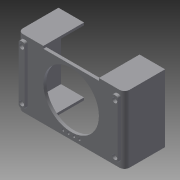
# Autodesk Inventor part: Enclosure01
Saved by Autodesk Inventor 2013 (Build 170138000, 138)
## iProperties
Created: 2014-04-13
Part Number: Enclosure01
Material: Generic
Document SubType Name: Modeling
Designer: spichelh
Density: 1 g/cm^3
Author: spichelh
Autodesk Inventor part; units mm, degrees
ref_plane "YZ Plane" through (0, 0, 0) normal (1, 0, 0) x (0, 1, 0)
ref_plane "XZ Plane" through (0, 0, 0) normal (0, 1, 0) x (-1, 0, 0)
ref_plane "XY Plane" through (0, 0, 0) normal (0, 0, 1) x (1, 0, 0)
sketch "Sketch1" plane through (0, 0, 0) normal (0, 0, 1) x (1, 0, 0)
  circle A0 centre (37.2069, 31.0185) radius 28
  line L0 (-13.5931, 3.1035) -> (88.0069, 3.1035) construction
  line L1 (14.2069, 60.2535) -> (-13.5931, 60.2535) construction
  line L2 (88.0069, 60.2535) -> (60.0869, 60.2535) construction
  line L3 (88.0069, 3.1035) -> (88.0069, 60.2535) construction
  line L4 (-13.5931, 60.2535) -> (-13.5931, 3.1035) construction
  line L5 (11.269, 60.2207) -> (67.149, 60.2207) construction
  line L6 (67.149, 60.2207) -> (67.149, 72.2207) construction
  line L7 (67.149, 72.2207) -> (11.269, 72.2207) construction
  line L8 (11.269, 72.2207) -> (11.269, 60.2207) construction
  circle A1 centre (61.389, 6.2635) radius 1.5 construction
  circle A2 centre (61.389, 55.7935) radius 1.5 construction
  circle A3 centre (5.509, 55.7935) radius 1.5 construction
  circle A4 centre (11.269, 6.9135) radius 1.5 construction
  arc A5 (11.269, 7.6907) -> (11.269, 1.6907) centre (11.269, 4.6907) ccw construction
  line L9 (11.269, 1.6907) -> (11.269, -3.7465) construction
  line L10 (11.269, -3.7465) -> (67.149, -3.7465) construction
  line L11 (67.149, -3.7465) -> (67.149, 1.6907) construction
  arc A6 (67.149, 1.6907) -> (67.149, 7.6907) centre (67.149, 4.6907) ccw construction
  line L12 (67.149, 7.6907) -> (67.149, 51.2207) construction
  arc A7 (67.149, 51.2207) -> (67.149, 57.2207) centre (67.149, 54.2207) ccw construction
  line L13 (67.149, 57.2207) -> (67.149, 60.2207) construction
  line L14 (67.149, 60.2207) -> (11.269, 60.2207) construction
  line L15 (11.269, 60.2207) -> (11.269, 57.2207) construction
  arc A8 (11.269, 57.2207) -> (11.269, 51.2207) centre (11.269, 54.2207) ccw construction
  line L16 (11.269, 51.2207) -> (11.269, 7.6907) construction
  line L17 (-16.5931, -3.7465) -> (91.0069, -3.7465)
  line L18 (91.0069, -3.7465) -> (91.0069, 64.2535)
  line L19 (91.0069, 64.2535) -> (-16.5931, 64.2535)
  line L20 (-16.5931, 64.2535) -> (-16.5931, -3.7465)
  line L21 (37.2069, -3.7465) -> (37.2069, 64.2535) construction
  circle A9 centre (37.2069, 31.0185) radius 23 projected
  point P0 (0, 0)
  dimension "d42" = 0
  dimension "d43" = 3
  dimension "d44" = 3
  dimension "d45" = 4
  dimension "d46" = 4
  dimension "d47" = 57.15
  dimension "d48" = 57.15
  dimension "d49" = 101.6
  dimension "d50" = 3.81
  dimension "d56" = 68
  dimension "d59" = 56
  constraints: 44 end point, 9 centre point, 8 point on circle, 2 midpoint, 2 parallel, 1 concentric, 1 horizontal, 1 perpendicular, 1 point on line
  measures "d42" distance between parallel lines of L17 L10
  measures "d43" distance between parallel lines of L4 L20
  measures "d44" distance between parallel lines of L18 L3
  measures "d45" distance between parallel lines of L19 L1
  measures "d46" distance between parallel lines of L19 L2
  measures "d47" distance between parallel lines of L0 L1
  measures "d48" distance between parallel lines of L2 L0
  measures "d49" distance between parallel lines of L4 L3
  measures "d50" distance from line of L0 A4.centre
  measures "d56" distance between parallel lines of L19 L17
  measures "d59" diameter of A0
extrude "Extrusion1" add sketch "Sketch1" along normal blind 3 contours L20 L19 L18 L17
sketch "Sketch2" plane through (0, 0, 0) normal (0, 0, -1) x (-1, 0, 0)
  circle A0 centre (-37.2069, 31.0185) radius 28 projected
  line L0 (16.5931, -3.7465) -> (-91.0069, -3.7465) projected
  line L1 (16.5931, 64.2535) -> (16.5931, -3.7465) projected
  line L2 (-91.0069, 64.2535) -> (16.5931, 64.2535) projected
  line L3 (-91.0069, -3.7465) -> (-91.0069, 64.2535) projected
  line L4 (-88.5069, 61.7535) -> (14.0931, 61.7535)
  line L5 (14.0931, 61.7535) -> (14.0931, -1.2465)
  line L6 (14.0931, -1.2465) -> (-88.5069, -1.2465)
  line L7 (-88.5069, -1.2465) -> (-88.5069, 61.7535)
  dimension "d51" = 2.5
  dimension "d52" = 2.5
  dimension "d53" = 2.5
  dimension "d54" = 2.5
  constraints: 8 end point, 2 parallel, 1 horizontal, 1 perpendicular
  measures "d51" distance between parallel lines of L4 L2
  measures "d52" distance between parallel lines of L3 L7
  measures "d53" distance between parallel lines of L1 L5
  measures "d54" distance between parallel lines of L0 L6
extrude "Extrusion2" add sketch "Sketch2" along normal blind 38 contours L0 L3 L2 L1
sketch "Sketch4" plane through (0, 0, 3) normal (0, 0, 1) x (1, 0, 0)
  circle A0 centre (-9.7831, 55.7835) radius 1.4 projected
  circle A1 centre (-9.7831, 6.2535) radius 1.4 projected
  circle A2 centre (84.1969, 6.2535) radius 1.4 projected
  circle A3 centre (84.1969, 55.7835) radius 1.4 projected
  point P0 (0, 0)
extrude "Extrusion3" cut sketch "Sketch4" against normal blind 3
chamfer "Chamfer1" [suppressed]
sketch "Sketch5" plane through (-16.5931, 64.2535, 3) normal (0, 1, 0) x (1, 0, 0)
  line L0 (0, 0) -> (107.6, 0)
  line L1 (25.8, 63) -> (81.8, 63)
  line L2 (81.8, 63) -> (81.8, 7)
  line L3 (81.8, 7) -> (25.8, 7)
  line L4 (25.8, 7) -> (25.8, 63)
  line L5 (53.8, 0) -> (53.8, -31.7336) construction
  line L6 (25.8, 63) -> (81.8, 7) construction
  line L7 (81.8, 63) -> (25.8, 7) construction
  line L8 (104.9242, 0) -> (-0.6758, 0)
  line L9 (107.6, 0) -> (0, 0) projected
  line L10 (0, 41) -> (107.6, 41) projected
  line L11 (53.8, 41) -> (53.8, 0) construction
  point P0 (19.351, -30)
  point P1 (53.8, 35)
  point P2 (53.8, 35)
  dimension "d28" = 56
  dimension "d29" = 56
  dimension "d41" = 7
  constraints: 20 end point, 5 midpoint, 3 parallel, 2 point on line, 1 collinear, 1 horizontal, 1 perpendicular
  measures "d28" distance of L2.end L3.end
  measures "d29" distance of L1.end L2.end
  measures "d41" distance between parallel lines of L8 L3
extrude "Extrusion4" cut sketch "Sketch5" against normal blind 100
fillet "Fillet2" radius 5 2 edges at (-16.5931, 30.2535, 3) (91.0069, 30.2535, 3)
fillet "Fillet3" radius 5 2 edges at (-14.0931, 30.2535, 0) (88.5069, 30.2535, 0)
sketch "Sketch6" plane through (9.2069, 64.2535, -4) normal (0, 1, 0) x (1, 0, 0)
  line L0 (76.8, -7) -> (-20.8, -7) projected
  line L1 (0, 0) -> (56, 0)
  line L2 (56, 0) -> (56, -7)
  line L3 (56, -7) -> (0, -7)
  line L4 (0, -7) -> (0, 0)
  point P0 (-9.2069, -4)
  constraints: 8 end point, 2 parallel, 1 horizontal, 1 perpendicular, 1 point on line
extrude "Extrusion5" cut sketch "Sketch6" against normal blind 2.5
sketch "Sketch7" plane through (0, 0, 3) normal (0, 0, 1) x (1, 0, 0)
  line L0 (-11.5931, -3.7465) -> (86.0069, -3.7465) projected
  line L1 (65.2069, 61.7535) -> (9.2069, 61.7535) projected
  line L2 (37.2069, -3.7465) -> (37.2069, 61.7535) construction
  line L3 (23.1969, -0.7465) -> (23.1969, -0.7465)
  line L4 (22.1969, 0.2535) -> (22.1969, 1.2535)
  line L5 (23.1969, 2.2535) -> (23.1969, 2.2535)
  line L6 (24.1969, 1.2535) -> (24.1969, 0.2535)
  arc A0 (24.1969, 1.2535) -> (23.1969, 2.2535) centre (23.1969, 1.2535) ccw
  arc A1 (23.1969, 2.2535) -> (22.1969, 1.2535) centre (23.1969, 1.2535) ccw
  arc A2 (22.1969, 0.2535) -> (23.1969, -0.7465) centre (23.1969, 0.2535) ccw
  arc A3 (23.1969, -0.7465) -> (24.1969, 0.2535) centre (23.1969, 0.2535) ccw
  line L7 (27.6969, 0.2535) -> (27.6969, 1.2535)
  line L8 (29.6969, 1.2535) -> (29.6969, 0.2535)
  arc A4 (29.6969, 1.2535) -> (28.6969, 2.2535) centre (28.6969, 1.2535) ccw
  arc A5 (28.6969, 2.2535) -> (27.6969, 1.2535) centre (28.6969, 1.2535) ccw
  arc A6 (27.6969, 0.2535) -> (28.6969, -0.7465) centre (28.6969, 0.2535) ccw
  arc A7 (28.6969, -0.7465) -> (29.6969, 0.2535) centre (28.6969, 0.2535) ccw
  line L9 (44.7169, 0.2535) -> (44.7169, 1.2535)
  line L10 (46.7169, 1.2535) -> (46.7169, 0.2535)
  arc A8 (46.7169, 1.2535) -> (45.7169, 2.2535) centre (45.7169, 1.2535) ccw
  arc A9 (45.7169, 2.2535) -> (44.7169, 1.2535) centre (45.7169, 1.2535) ccw
  arc A10 (44.7169, 0.2535) -> (45.7169, -0.7465) centre (45.7169, 0.2535) ccw
  arc A11 (45.7169, -0.7465) -> (46.7169, 0.2535) centre (45.7169, 0.2535) ccw
  line L11 (38.6969, 0.2535) -> (38.6969, 1.2535)
  line L12 (40.6969, 1.2535) -> (40.6969, 0.2535)
  arc A12 (40.6969, 1.2535) -> (39.6969, 2.2535) centre (39.6969, 1.2535) ccw
  arc A13 (39.6969, 2.2535) -> (38.6969, 1.2535) centre (39.6969, 1.2535) ccw
  arc A14 (38.6969, 0.2535) -> (39.6969, -0.7465) centre (39.6969, 0.2535) ccw
  arc A15 (39.6969, -0.7465) -> (40.6969, 0.2535) centre (39.6969, 0.2535) ccw
  line L13 (29.6969, 0.7535) -> (44.7169, 0.7535) construction
  point P0 (0, 0)
  point P1 (24.1969, -0.7465)
  point P2 (22.1969, 2.2535)
  point P3 (24.1969, 2.2535)
  point P4 (29.6969, -0.7465)
  point P5 (27.6969, 2.2535)
  point P6 (29.6969, 2.2535)
  point P7 (46.7169, -0.7465)
  point P8 (44.7169, 2.2535)
  point P9 (46.7169, 2.2535)
  point P10 (40.6969, -0.7465)
  point P11 (38.6969, 2.2535)
  point P12 (40.6969, 2.2535)
  point P13 (37.2069, 0.7535)
  dimension "d64" = 2
  dimension "d66" = 3
  dimension "d67" = 1
  dimension "d68" = 1
  dimension "d69" = 4
  dimension "d78" = 16.5
  dimension "d79" = 13.01
  dimension "d80" = 1.49
  constraints: 32 point on circle, 24 end point, 16 centre point, 16 point on line, 8 tangent, 5 midpoint, 2 equal radius, 2 parallel, 1 horizontal, 1 perpendicular
  measures "d64" distance of point (22.197, 2.253) point (24.197, 2.253)
  measures "d66" distance of point (24.197, 2.253) point (24.197, -0.747)
  measures "d67" radius of A0
  measures "d68" radius of A3
  measures "d69" distance from line of L0 A3.centre
  measures "d78" distance of A14.centre A3.centre
  measures "d79" distance from line of L6 point (37.207, 0.753)
  measures "d80" distance from line of point (37.207, 0.753) L11
extrude "Extrusion6" cut sketch "Sketch7" against normal blind 3
sketch "Sketch10" plane through (0, 0, 3) normal (0, 0, 1) x (1, 0, 0)
  circle A0 centre (37.2069, 31.0185) radius 28 projected
  circle A1 centre (84.1969, 55.7835) radius 1.4 projected
  circle A2 centre (-9.7831, 6.2535) radius 1.4 projected
  circle A3 centre (-9.7831, 55.7835) radius 1.4 projected
  circle A4 centre (84.1969, 6.2535) radius 1.4 projected
  line L0 (-8.7831, 60.1835) -> (-10.7831, 60.1835)
  line L1 (-12.7831, 58.1835) -> (-12.7831, 3.8535)
  line L2 (-10.7831, 1.8535) -> (-8.7831, 1.8535)
  line L3 (-6.7831, 3.8535) -> (-6.7831, 58.1835)
  arc A5 (-6.7831, 58.1835) -> (-8.7831, 60.1835) centre (-8.7831, 58.1835) ccw
  arc A6 (-10.7831, 60.1835) -> (-12.7831, 58.1835) centre (-10.7831, 58.1835) ccw
  arc A7 (-8.7831, 1.8535) -> (-6.7831, 3.8535) centre (-8.7831, 3.8535) ccw
  arc A8 (-12.7831, 3.8535) -> (-10.7831, 1.8535) centre (-10.7831, 3.8535) ccw
  line L4 (37.2069, 31.0185) -> (37.2069, 47.569) construction
  line L5 (83.1969, 60.1835) -> (85.1969, 60.1835)
  line L6 (87.1969, 58.1835) -> (87.1969, 3.8535)
  line L7 (85.1969, 1.8535) -> (83.1969, 1.8535)
  line L8 (81.1969, 3.8535) -> (81.1969, 58.1835)
  arc A9 (83.1969, 60.1835) -> (81.1969, 58.1835) centre (83.1969, 58.1835) ccw
  arc A10 (87.1969, 58.1835) -> (85.1969, 60.1835) centre (85.1969, 58.1835) ccw
  arc A11 (81.1969, 3.8535) -> (83.1969, 1.8535) centre (83.1969, 3.8535) ccw
  arc A12 (85.1969, 1.8535) -> (87.1969, 3.8535) centre (85.1969, 3.8535) ccw
  point P0 (0, 0)
  dimension "d101" = 3
  dimension "d103" = 3
  dimension "d104" = 3
  dimension "d105" = 3
  dimension "d106" = 2
  dimension "d107" = 2
  constraints: 18 end point, 16 point on circle, 12 symmetric about line, 8 centre point, 8 tangent, 3 parallel, 2 equal radius, 1 horizontal, 1 perpendicular, 4 other
  measures "d101" distance edge to line of A2 L2
  measures "d103" distance edge to line of A3 L0
  measures "d104" distance from line of L1 A2.centre
  measures "d105" distance from line of L3 A3.centre
  measures "d106" radius of A5
  measures "d107" radius of A6
extrude "Extrusion9" add sketch "Sketch10" along normal blind 3 and the other way blind 2 contours A5 L3 A7 L2 A8 L1 A6 L0 | L5 A10 L6 A12 L7 A11 L8 A9
sketch "Sketch11" plane through (0, 0, 6) normal (0, 0, 1) x (1, 0, 0)
  circle A0 centre (-9.7831, 55.7835) radius 1.4 projected
  circle A1 centre (-9.7831, 6.2535) radius 1.4 projected
  line L0 (81.1969, 58.1835) -> (81.1969, 3.8535) projected
  arc A2 (81.1969, 3.8535) -> (83.1969, 1.8535) centre (83.1969, 3.8535) ccw projected
  line L1 (83.1969, 1.8535) -> (85.1969, 1.8535) projected
  arc A3 (85.1969, 1.8535) -> (87.1969, 3.8535) centre (85.1969, 3.8535) ccw projected
  line L2 (87.1969, 3.8535) -> (87.1969, 58.1835) projected
  arc A4 (87.1969, 58.1835) -> (85.1969, 60.1835) centre (85.1969, 58.1835) ccw projected
  line L3 (85.1969, 60.1835) -> (83.1969, 60.1835) projected
  arc A5 (83.1969, 60.1835) -> (81.1969, 58.1835) centre (83.1969, 58.1835) ccw projected
  circle A6 centre (-9.7831, 55.7835) radius 2.5
  circle A7 centre (-9.7831, 6.2535) radius 2.5
  circle A8 centre (78.5569, 55.7835) radius 2.5
  circle A9 centre (78.5569, 6.2535) radius 2.5
  point P0 (0, 0)
  dimension "d112" = 5
  dimension "d114" = 5
  dimension "d115" = 5
  dimension "d116" = 5
  constraints: 4 centre point
  measures "d112" diameter of A6
  measures "d114" diameter of A7
  measures "d115" diameter of A8
  measures "d116" diameter of A9
extrude "Extrusion10" cut sketch "Sketch11" against normal blind 3 contours A0 | A1 | A6 | A7 | A8 | A9
body "Solid1"
